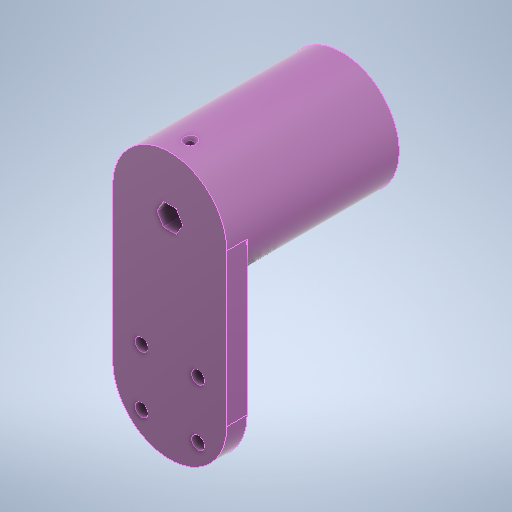
# Autodesk Inventor part: pen_holder
Saved by Autodesk Inventor 2025.1 (Build 291241000, 241)
## iProperties
Created: 2024-08-22
Part Number: pen_holder
Material: LCP Plastic
Document SubType Name: Modeling
Designer: pedro
Density: 1.626 g/cm^3
Appearance: Smooth - Purple
Author: pedro
Autodesk Inventor part; units mm, degrees
ref_plane "YZ Plane" through (0, 0, 0) normal (1, 0, 0) x (0, 1, 0)
ref_plane "XZ Plane" through (0, 0, 0) normal (0, 1, 0) x (-1, 0, 0)
ref_plane "XY Plane" through (0, 0, 0) normal (0, 0, 1) x (1, 0, 0)
sketch "Sketch1" plane through (0, 0, 0) normal (0, 0, 1) x (1, 0, 0)
  arc A0 (-22.5, 0) -> (22.5, 0) centre (0, 0) ccw
  circle A1 centre (-11.14, 11.14) radius 2.5
  circle A2 centre (-11.14, -11.14) radius 2.5
  circle A3 centre (11.14, -11.14) radius 2.5
  circle A4 centre (11.14, 11.14) radius 2.5
  line L0 (-22.5, 0) -> (-22.5, 60)
  arc A5 (22.5, 60) -> (-22.5, 60) centre (0, 60) ccw
  line L1 (22.5, 60) -> (22.5, 0)
  dimension "d0" = 45
  dimension "d3" = 5
  dimension "d4" = 11.14
  dimension "d5" = 11.14
  dimension "d8" = 360
  dimension "d12" = 60
  dimension "d27" = 60
  dimension "d28" = 60
  constraints: 6 centre point, 4 end point, 4 point on circle, 2 vertical, 1 coincident, 9 other
  measures "d0" diameter of A0
  measures "d3" diameter of A1
  measures "d4" horizontal distance of A0.centre A1.centre
  measures "d5" horizontal distance of A0.centre A1.centre
  measures "d12" distance of L0.start L0.end
  measures "d27" distance of L1.start L1.end
  measures "d28" distance of A0.centre A5.centre
extrude "Extrusion1" add sketch "Sketch1" along normal blind 8
sketch "Sketch2" plane through (0, 0, 0) normal (0, 0, -1) x (-1, 0, 0)
  arc A0 (22.5, 60) -> (-22.5, 60) centre (0, 60) ccw projected
  circle A1 centre (0, 60) radius 22.5
  line L0 (5, 60) -> (2.5, 55.6699)
  line L1 (2.5, 55.6699) -> (-2.5, 55.6699)
  line L2 (-2.5, 55.6699) -> (-5, 60)
  line L3 (-5, 60) -> (-2.5, 64.3301)
  line L4 (-2.5, 64.3301) -> (2.5, 64.3301)
  line L5 (2.5, 64.3301) -> (5, 60)
  point P0 (0, 0)
  dimension "d14" = 10
  constraints: 12 end point, 2 coincident, 1 centre point, 13 other
  measures "d14" distance of L2.end L0.start
extrude "Extrusion2" add sketch "Sketch2" along normal blind 60
thicken "Thicken1" operation cut thickness 20 both sides no extend neighbours no toward (0, 0, 1) faces at (-0.8333, 58.5566, 0)
ref_plane "Work Plane1" through (0, 82.5, 8) normal (0, 1, 0) x (-1, 0, 0)
sketch "Sketch4" plane through (0, 82.5, 8) normal (0, 1, 0) x (-1, 0, 0)
  line L0 (22.5, -8) -> (-22.5, -8) projected
  circle A0 centre (0, -8) radius 1.5
  dimension "d19" = 3
  constraints: 1 centre point, 1 midpoint
  measures "d19" diameter of A0
hole "Hole1" at (0, 82.5, 0) direction (0, -1, 0) diameter 3 depth 18.5 countersink diameter 5 countersink angle 82
equation "\"d12\" = d27"
equation "\"d28\" = d27"
body "Solid1"
